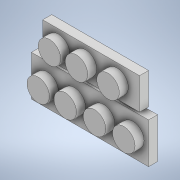
# Autodesk Inventor part: Push Buttons
Saved by Autodesk Inventor 2021 (Build 250183000, 183)
## iProperties
Created: 2021-07-28
Part Number: Push Buttons
Material: Generic
Document SubType Name: Modeling
Designer: USER
Density: 1 g/cm^3
Appearance: Default
Author: USER
Autodesk Inventor part; units mm, degrees
ref_plane "YZ Plane" through (0, 0, 0) normal (1, 0, 0) x (0, 1, 0)
ref_plane "XZ Plane" through (0, 0, 0) normal (0, 1, 0) x (-1, 0, 0)
ref_plane "XY Plane" through (0, 0, 0) normal (0, 0, 1) x (1, 0, 0)
sketch "Sketch1" plane through (0, 0, 0) normal (0, 0, 1) x (1, 0, 0)
  line L0 (4, 18) -> (56, 18)
  line L1 (56, 18) -> (56, 0)
  line L2 (56, 0) -> (4, 0)
  line L3 (4, 0) -> (4, 18)
  point P0 (0, 0)
  constraints: 8 end point, 2 parallel, 1 horizontal, 1 perpendicular
extrude "Extrusion1" add sketch "Sketch1" against normal blind 4
sketch "Sketch2" plane through (0, 0, 0) normal (0, 0, 1) x (1, 0, 0)
  circle A0 centre (11, 9) radius 5
  circle A1 centre (23, 9) radius 5
  circle A2 centre (36, 9) radius 5
  circle A3 centre (49, 9) radius 5
  point P0 (0, 0)
  constraints: 4 centre point
sketch "Sketch3" plane through (0, 0, 0) normal (0, 0, 1) x (1, 0, 0)
  line L0 (9, 33) -> (52, 33)
  line L1 (52, 33) -> (52, 19)
  line L2 (52, 19) -> (9, 19)
  line L3 (9, 19) -> (9, 33)
  point P0 (0, 0)
  constraints: 8 end point, 2 parallel, 1 horizontal, 1 perpendicular
extrude "Extrusion2" add sketch "Sketch3" against normal blind 4
sketch "Sketch4" plane through (0, 0, 0) normal (0, 0, 1) x (1, 0, 0)
  circle A0 centre (16, 26) radius 5
  circle A1 centre (28, 26) radius 5
  circle A2 centre (42, 26) radius 5
  point P0 (0, 0)
  constraints: 3 centre point
extrude "Extrusion3" add sketch "Sketch2" along normal blind 4
extrude "Extrusion4" add sketch "Sketch4" along normal blind 4
body "Solid1"
